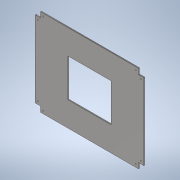
# Autodesk Inventor part: Chapa-0001-001
Saved by Autodesk Inventor 2020.1 (Build 241239000, 239)
## iProperties
Created: 2024-04-12
Part Number: Chapa-0001-001
Material: Steel, Galvanized
Document SubType Name: Sheet Metal
Designer: MiguelBarbosa
Density: 7.85 g/cm^3
Sheet Metal Rule: Default_mm
Appearance: Galvanized
Author: MiguelBarbosa
Autodesk Inventor part; units mm, degrees
ref_plane "YZ Plane" through (0, 0, 0) normal (1, 0, 0) x (0, 1, 0)
ref_plane "XZ Plane" through (0, 0, 0) normal (0, 1, 0) x (-1, 0, 0)
ref_plane "XY Plane" through (0, 0, 0) normal (0, 0, 1) x (1, 0, 0)
sketch "Sketch3" plane through (0, 0, 0) normal (0, 0, 1) x (1, 0, 0)
  line L0 (-500, -400) -> (500, -400)
  line L1 (500, -400) -> (500, 400)
  line L2 (500, 400) -> (-500, 400)
  line L3 (-500, 400) -> (-500, -400)
  line L4 (-500, -400) -> (500, 400) construction
  line L5 (500, -400) -> (-500, 400) construction
  point P0 (0, 0)
  dimension "d9" = 1000
  dimension "d10" = 800
  measures "d9" distance of L1.end L2.end
  measures "d10" distance of L2.end L0.start
extrude "Plate2" add sketch "Sketch3" along normal mid plane 10
sketch "Sketch4" plane through (0, 0, 5) normal (0, 0, 1) x (1, 0, 0)
  line L0 (-200, -175) -> (200, -175)
  line L1 (200, -175) -> (200, 175)
  line L2 (200, 175) -> (-200, 175)
  line L3 (-200, 175) -> (-200, -175)
  line L4 (-200, -175) -> (200, 175) construction
  line L5 (200, -175) -> (-200, 175) construction
  point P0 (0, 0)
  dimension "d12" = 400
  dimension "d13" = 350
  constraints: 12 end point, 2 midpoint, 2 parallel, 1 horizontal, 1 perpendicular
  measures "d12" distance of L1.end L2.end
  measures "d13" distance of L2.end L0.start
extrude "Cut2" cut sketch "Sketch4" against normal blind 10
sketch "Sketch7" plane through (0, 0, 5) normal (0, 0, 1) x (1, 0, 0)
  line L0 (-450, 400) -> (-500, 400)
  line L1 (-500, 400) -> (-500, 350)
  line L2 (-500, 350) -> (-450, 350)
  line L3 (-450, 350) -> (-450, 400)
  line L4 (-450, 400) -> (-500, 350) construction
  line L5 (-500, 400) -> (-450, 350) construction
  circle A0 centre (-425, 375) radius 5.1
  circle A1 centre (-475, 325) radius 5.1
  point P0 (0, 0)
  point P1 (-475, 375)
  point P2 (-475, 375)
  point P3 (-475, 375)
  dimension "d20" = 50
  dimension "d21" = 50
  dimension "d26" = 10.2
  dimension "d27" = 25
  dimension "d28" = 25
  constraints: 12 end point, 4 midpoint, 2 centre point, 2 parallel, 1 coincident, 1 equal radius, 1 horizontal, 1 horizontal alignment, 1 perpendicular, 1 vertical alignment
  measures "d20" distance of L1.end L2.end
  measures "d21" distance of L2.end L0.start
  measures "d26" diameter of A0
  measures "d27" distance from line of L3 A0.centre
  measures "d28" distance from line of A1.centre L2
extrude "Cut4" cut sketch "Sketch7" against normal blind 10
mirror "Mirror5" about plane through (0, 0, 0) normal (0, 1, 0) of "Cut4"
mirror "Mirror6" about plane through (0, 0, 0) normal (1, 0, 0) of "Cut4", "Mirror5"
equation "\"d14\" = Thickness"
equation "\"d21\" = d20"
equation "\"d28\" = d27"
equation "\"d22\" = Thickness"
equation "\"d11\" = Thickness"
equation "\"BendReliefDepth\" = 0.5 * Thickness"
equation "\"Thickness\" = 10"
body "Solid2"
